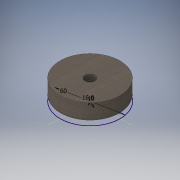
# Autodesk Inventor part: Foot
Saved by Autodesk Inventor 2018.2 (Build 222227000, 227)
## iProperties
Created: 2018-03-10
Part Number: Foot
Material: Generisch
Document SubType Name: Modeling
Designer: JochenAlt
Density: 1 g/cm^3
Appearance: Vorgabe
Author: JochenAlt
Autodesk Inventor part; units mm, degrees
ref_plane "YZ Plane" through (0, 0, 0) normal (1, 0, 0) x (0, 1, 0)
ref_plane "XZ Plane" through (0, 0, 0) normal (0, 1, 0) x (-1, 0, 0)
ref_plane "XY Plane" through (0, 0, 0) normal (0, 0, 1) x (1, 0, 0)
sketch "Skizze1" plane through (0, 0, 0) normal (0, 0, 1) x (1, 0, 0)
  line L0 (0, 42) -> (0, -42) construction
  line L1 (-42, 0) -> (42, 0) construction
  circle A0 centre (0, 0) radius 30
  circle A1 centre (0, 0) radius 8.3
  circle A2 centre (0, 0) radius 5
  dimension "d0" = 60
  dimension "d1" = 16.6
  dimension "d2" = 10
  constraints: 3 centre point, 3 coincident
  measures "d0" diameter of A0
  measures "d1" diameter of A1
  measures "d2" diameter of A2
extrude "Extrusion1" add sketch "Skizze1" along normal blind 20 contours A0
thread "Gewinde2" size "M16x2" class "6H" standard "ANSI Metric M Profile" length 15
sketch "Skizze7" plane through (0, 0, 0) normal (1, 0, 0) x (0, 1, 0)
  line L0 (8.3, 0) -> (8.3, 15)
  line L1 (8.3, 15) -> (6.9948, 15)
  line L2 (6.9948, 15) -> (6.9948, 0)
  line L3 (6.9948, 0) -> (8.3, 0)
  line L4 (0, -6.6391) -> (0, 24.4398) projected
  constraints: 8 end point
revolve "Umdrehung3" add sketch "Skizze7" angle 360 about axis through (0, 0, 0) along (0, 0, 1) separate body
sketch "Skizze6" plane through (0, 8.3, 0) normal (-1, 0, 0) x (0, 0, 1)
  line L0 (-1.1849, -0.1069) -> (-1.0001, -0.1069) construction
  line L1 (0.1847, -1.1986) -> (-0.0001, -1.5188) construction
  line L2 (-2.0001, -1.5188) -> (-2.185, -1.1986) construction
  line L3 (-0.8153, -0.1069) -> (-1.0001, 0.2133) construction
  line L4 (-1.0001, 0.2133) -> (-1.1849, -0.1069) construction
  line L5 (-2.0001, -1.5188) -> (-1.8153, -1.1986) construction
  line L6 (-0.8153, -0.1069) -> (-0.1849, -1.1986)
  line L7 (-2.185, -1.1986) -> (-1.8153, -1.1986) construction
  arc A0 (-2.185, -1.1986) -> (-2.0001, -1.3053) centre (-2.0001, -1.0919) ccw construction
  line L8 (0.1847, -1.1986) -> (-0.1849, -1.1986) construction
  line L9 (-2.0001, -1.5188) -> (-2.0001, -1.1986) construction
  line L10 (-0.0001, -1.5188) -> (-0.0001, -1.1986) construction
  line L11 (-1.0001, 0.2133) -> (-1.0001, -0.0002) construction
  line L12 (-2.0001, -1.3053) -> (-0.0001, -1.3053)
  arc A1 (-2.0001, -1.3053) -> (-1.8153, -1.1986) centre (-2.0001, -1.0919) ccw
  line L13 (-0.1849, -1.1986) -> (-0.0001, -1.5188) construction
  line L14 (-1.8153, -1.1986) -> (-1.1849, -0.1069)
  line L15 (-0.0001, -0.0002) -> (-0.0001, 0.0177)
  line L16 (-0.0001, 0.0177) -> (-0.0001, -0.0002)
  line L17 (-0.0001, -0.0002) -> (0.0334, -0.0002)
  arc A2 (-0.1849, -1.1986) -> (-0.0001, -1.3053) centre (-0.0001, -1.0919) ccw
  arc A3 (-0.0001, -1.3053) -> (0.1847, -1.1986) centre (-0.0001, -1.0919) ccw construction
  arc A4 (-1.0001, -0.0002) -> (-1.1849, -0.1069) centre (-1.0001, -0.2136) ccw
  arc A5 (-0.8153, -0.1069) -> (-1.0001, -0.0002) centre (-1.0001, -0.2136) ccw
  line L18 (-1.0001, -0.0002) -> (-1.0001, -0.1069) construction
  line L19 (-1.0001, -0.1069) -> (-0.8153, -0.1069) construction
  dimension "d49" = 60
  dimension "d50" = 0.3202
  dimension "d51" = 0.3202
  dimension "Skizze6_ThreadOffset" = 0
  dimension "Skizze6_MajorRadius" = 1.3052
  dimension "d54" = 2
  dimension "Skizze6_MinorRadius" = 0
  constraints: 40 end point, 12 point on circle, 10 parallel, 8 tangent, 6 centre point, 6 collinear, 2 midpoint, 2 point on line, 1 horizontal, 1 perpendicular, 3 other
  measures "d49" angle of L6 L14
  measures "d50" distance of L3.end L0.end
  measures "d51" distance of L1.end L10.end
  measures "Skizze6_ThreadOffset" distance between parallel lines of L15 L10
  measures "Skizze6_MajorRadius" distance from line of L12 L15.start
  measures "d54" distance from line of L1.end L9
  measures "Skizze6_MinorRadius" distance edge to line of A5 L17
coil "Spirale3" sketch "Skizze6" operation cut axis through (0, 0, 0) along (0, 0, 1) pitch 2.002 turns 9.490509 hand right bodies 2
combine bodies "Kombinieren2" operation type add bodies to combine 1 2
chamfer "Fase1" distance 20 distance2 4 1 edges at (-30, 0, 0) measured on face at (-29.5, 0, 0)
fillet "Rundung1" radius 2 1 edges at (-30, 0, 4)
extrude "Extrusion2" add sketch "Skizze1" against normal up to surface (5 mm away) from surface at 20 contours A1 bodies 1
equation "\"d49\" = d56"
equation "\"d50\" = 0.160083 * Skizze6_Pitch"
equation "\"d51\" = 0.160083 * Skizze6_Pitch"
equation "\"d54\" = Skizze6_Pitch"
equation "\"d14\" = 60deg"
equation "\"Skizze2_Pitch\" = 2"
equation "\"d34\" = 60deg"
equation "\"Skizze4_Pitch\" = 2"
equation "\"d56\" = 60deg"
equation "\"Skizze6_Pitch\" = 2"
